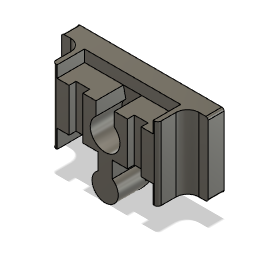
Duplo_Eisenbahn_adapter (Autodesk Fusion 360 design; units mm, degrees)
Autodesk Fusion 360 part; units mm, degrees
note: some values were not read from the file. Set by a fixed rule: which sketch regions a step uses.
sketch "Skizze1" plane through (0, 0, 0) normal (0, 0, 1) x (1, 0, 0)
  line L0 (32, 16) -> (-32, 16)
  line L1 (-32, 16) -> (-32, -16)
  line L2 (-32, -16) -> (32, -16)
  line L3 (32, -16) -> (32, 16)
  line L4 (32, 16) -> (-32, -16) construction
  line L5 (-32, 16) -> (32, -16) construction
  dimension "d1" = 64
  dimension "d2" = 32
  constraint horizontal L0
  constraint perpendicular L0 L1
  constraint parallel L0 L2
  constraint parallel L1 L3
  constraint coincident L4 origin
  constraint coincident L5 origin
  measures "d1" distance of L1.end L2.end
  measures "d2" distance of L0.end L1.end
extrude "Extrusion1" add sketch "Skizze1" along normal blind 20
sketch "Skizze2" plane through (0, 0, 0) normal (0, 0, -1) x (-1, 0, 0)
  line L0 (-32, 16) -> (-32, -16)
  line L1 (-32, -16) -> (32, -16)
  line L2 (32, -16) -> (32, 16)
  line L3 (32, 16) -> (-32, 16)
  line L4 (30.25, 14.25) -> (-30.25, 14.25)
  line L5 (-30.25, 14.25) -> (-30.25, -14.25)
  line L6 (-30.25, -14.25) -> (30.25, -14.25)
  line L7 (30.25, -14.25) -> (30.25, 14.25)
  line L8 (30.25, 14.25) -> (-30.25, -14.25) construction
  line L9 (-30.25, 14.25) -> (30.25, -14.25) construction
  line L10 (-25, 14.25) -> (-23.5, 14.25)
  line L11 (-23.5, 14.25) -> (-23.5, 12.75)
  line L12 (-23.5, 12.75) -> (-25, 12.75)
  line L13 (-25, 12.75) -> (-25, 14.25)
  line L14 (-30.25, 9) -> (-28.75, 9)
  line L15 (-28.75, 9) -> (-28.75, 7.5)
  line L16 (-28.75, 7.5) -> (-30.25, 7.5)
  line L17 (-30.25, 7.5) -> (-30.25, 9)
  line L18 (-10, 14.25) -> (-8.5, 14.25)
  line L19 (-8.5, 14.25) -> (-8.5, 12.75)
  line L20 (-8.5, 12.75) -> (-10, 12.75)
  line L21 (-10, 12.75) -> (-10, 14.25)
  line L22 (-24.25, 12.75) -> (-24.25, 14.25) construction
  line L23 (-28.75, 8.25) -> (-30.25, 8.25) construction
  line L24 (-9.25, 12.75) -> (-9.25, 14.25) construction
  line L25 (0, 0) -> (0, 14.25) construction
  line L26 (0, 0) -> (-30.25, 0) construction
  line L27 (24.25, 12.75) -> (24.25, 14.25) construction
  line L28 (8.5, 14.25) -> (8.5, 12.75)
  line L29 (28.75, 7.5) -> (30.25, 7.5)
  line L30 (10, 14.25) -> (8.5, 14.25)
  line L31 (8.5, 12.75) -> (10, 12.75)
  line L32 (23.5, 12.75) -> (25, 12.75)
  line L33 (28.75, 8.25) -> (30.25, 8.25) construction
  line L34 (28.75, 9) -> (28.75, 7.5)
  line L35 (25, 12.75) -> (25, 14.25)
  line L36 (30.25, 7.5) -> (30.25, 9)
  line L37 (9.25, 12.75) -> (9.25, 14.25) construction
  line L38 (30.25, 9) -> (28.75, 9)
  line L39 (10, 12.75) -> (10, 14.25)
  line L40 (25, 14.25) -> (23.5, 14.25)
  line L41 (23.5, 14.25) -> (23.5, 12.75)
  line L42 (-25, -12.75) -> (-25, -14.25)
  line L43 (-28.75, -9) -> (-28.75, -7.5)
  line L44 (-30.25, -9) -> (-28.75, -9)
  line L45 (30.25, -14.25) -> (-30.25, -14.25)
  line L46 (-28.75, -8.25) -> (-30.25, -8.25) construction
  line L47 (25, -14.25) -> (23.5, -14.25)
  line L48 (-10, -14.25) -> (-8.5, -14.25)
  line L49 (23.5, -12.75) -> (25, -12.75)
  line L50 (-23.5, -14.25) -> (-23.5, -12.75)
  line L51 (32, -16) -> (-32, -16)
  line L52 (10, -12.75) -> (10, -14.25)
  line L53 (-9.25, -12.75) -> (-9.25, -14.25) construction
  line L54 (-28.75, -7.5) -> (-30.25, -7.5)
  line L55 (8.5, -12.75) -> (10, -12.75)
  line L56 (-10, -12.75) -> (-10, -14.25)
  line L57 (28.75, -8.25) -> (30.25, -8.25) construction
  line L58 (-25, -14.25) -> (-23.5, -14.25)
  line L59 (8.5, -14.25) -> (8.5, -12.75)
  line L60 (24.25, -12.75) -> (24.25, -14.25) construction
  line L61 (-23.5, -12.75) -> (-25, -12.75)
  line L62 (30.25, -9) -> (28.75, -9)
  line L63 (-8.5, -14.25) -> (-8.5, -12.75)
  line L64 (23.5, -14.25) -> (23.5, -12.75)
  line L65 (30.25, -7.5) -> (30.25, -9)
  line L66 (10, -14.25) -> (8.5, -14.25)
  line L67 (-24.25, -12.75) -> (-24.25, -14.25) construction
  line L68 (28.75, -9) -> (28.75, -7.5)
  line L69 (9.25, -12.75) -> (9.25, -14.25) construction
  line L70 (-8.5, -12.75) -> (-10, -12.75)
  line L71 (-30.25, -7.5) -> (-30.25, -9)
  line L72 (28.75, -7.5) -> (30.25, -7.5)
  line L73 (25, -12.75) -> (25, -14.25)
  circle A0 centre (0, 0) radius 6.575
  circle A1 centre (16, 0) radius 6.575
  circle A2 centre (-16, 0) radius 6.575
  circle A3 centre (-16, 0) radius 5.075
  circle A4 centre (0, 0) radius 5.075
  circle A5 centre (16, 0) radius 5.075
  point P0 (32, 16)
  point P1 (30.25, 14.25)
  point P2 (0, -14.25)
  point P3 (32, -16)
  point P4 (30.25, -14.25)
  dimension "d7" = 1.75
  dimension "d8" = 1.75
  dimension "d9" = 1.5
  dimension "d10" = 1.5
  dimension "d11" = 6
  dimension "d12" = 6
  dimension "d13" = 15
  dimension "d14" = 13.15
  dimension "d17" = 16
  dimension "d18" = 0
  dimension "d19" = 1.5
  constraint horizontal L4
  constraint perpendicular L4 L5
  constraint parallel L4 L6
  constraint parallel L5 L7
  constraint coincident L8 L25.start
  constraint coincident L9 L25.start
  constraint coincident L25.start L26.start
  constraint horizontal L10
  constraint vertical L11
  constraint horizontal L12
  constraint vertical L13
  constraint coincident L4 L10.start
  constraint horizontal L14
  constraint vertical L15
  constraint horizontal L16
  constraint vertical L17
  constraint coincident L5 L14.start
  constraint horizontal L18
  constraint vertical L19
  constraint horizontal L20
  constraint vertical L21
  constraint coincident L4 L18.start
  constraint collinear L12 L20
  constraint equal L13 L14
  constraint equal L12 L20
  constraint equal L12 L15
  constraint midpoint L12 L22.start
  constraint midpoint L10 L22.end
  constraint midpoint L15 L23.start
  constraint midpoint L17 L23.end
  constraint midpoint L20 L24.start
  constraint midpoint L18 L24.end
  constraint midpoint L4 L25.end
  constraint midpoint L5 L26.end
  constraint symmetric L0.start L25 P0
  constraint symmetric L4.end L25 P1
  constraint symmetric L10.start L25 L35.end
  constraint symmetric L10.end L25 L40.end
  constraint symmetric L11.end L25 L32.start
  constraint symmetric L12.end L25 L32.end
  constraint symmetric L14.start L25 L36.end
  constraint symmetric L14.end L25 L34.start
  constraint symmetric L15.end L25 L29.start
  constraint symmetric L16.end L25 L29.end
  constraint symmetric L18.start L25 L30.start
  constraint symmetric L18.end L25 L28.start
  constraint symmetric L19.end L25 L28.end
  constraint symmetric L20.end L25 L31.end
  constraint symmetric L22.start L25 L27.start
  constraint symmetric L22.end L25 L27.end
  constraint symmetric L23.start L25 L33.start
  constraint symmetric L23.end L25 L33.end
  constraint symmetric L24.start L25 L37.start
  constraint symmetric L24.end L25 L37.end
  constraint symmetric L0.start L26 L0.end
  constraint symmetric P0 L26 P3
  constraint symmetric P1 L26 P4
  constraint symmetric L4.end L26 L5.end
  constraint symmetric L10.start L26 L42.end
  constraint symmetric L10.end L26 L50.start
  constraint symmetric L11.end L26 L50.end
  constraint symmetric L12.end L26 L42.start
  constraint symmetric L14.start L26 L44.start
  constraint symmetric L14.end L26 L43.start
  constraint symmetric L15.end L26 L43.end
  constraint symmetric L16.end L26 L54.end
  constraint symmetric L18.start L26 L48.start
  constraint symmetric L18.end L26 L48.end
  constraint symmetric L19.end L26 L63.end
  constraint symmetric L20.end L26 L56.start
  constraint symmetric L22.start L26 L67.start
  constraint symmetric L22.end L26 L67.end
  constraint symmetric L23.start L26 L46.start
  constraint symmetric L23.end L26 L46.end
  constraint symmetric L24.start L26 L53.start
  constraint symmetric L24.end L26 L53.end
  constraint symmetric L25.end L26 P2
  constraint symmetric L26 L40.end L47.end
  constraint symmetric L26 L28.start L59.start
  constraint symmetric L26 L30.start L52.end
  constraint symmetric L26 L37.start L69.start
  constraint symmetric L26 L33.end L57.end
  constraint symmetric L26 L37.end L69.end
  constraint symmetric L26 L29.end L65.start
  constraint symmetric L26 L29.start L68.end
  constraint symmetric L26 P0 P3
  constraint symmetric L26 L36.end L62.start
  constraint symmetric L26 L34.start L62.end
  constraint symmetric L26 L28.end L55.start
  constraint symmetric L26 L33.start L57.start
  constraint symmetric L26 L27.end L60.end
  constraint symmetric L26 L27.start L60.start
  constraint symmetric L26 L31.end L52.start
  constraint symmetric L26 L32.start L49.start
  constraint symmetric L26 L32.end L49.end
  constraint symmetric L26 L35.end L47.start
  constraint symmetric L26 P1 P4
  constraint concentric A2 A3
  constraint concentric A1 A5
  constraint equal A4 A5
  constraint equal A3 A4
  measures "d7" distance of L3 L4
  measures "d8" distance of L0 L5
  measures "d9" distance of L10.end L11.end
  measures "d10" distance of L11.end L12.end
  measures "d11" distance of L4 L23
  measures "d12" distance of L5 L22
  measures "d13" distance of L22 L24
  measures "d14" diameter of A0
  measures "d19" distance of A1 A5
extrude "Extrusion2" cut sketch "Skizze2" against normal blind 5 contours L4 L5 L6 L7 L11 L12 L13 L14 L15 L16 L19 L20 L21 L28 L29 L31 L32 L34 L35 L38 L39 L41 L42 L43 L44 L45 L49 L50 L52 L54 L55 L56 L59 L61 L62 L63 L64 L68 L70 L72 L73 | A3 | A4 | A5
sketch "Skizze3" plane through (0, 0, 20) normal (0, 0, 1) x (1, 0, 0)
  line L0 (32, -16) -> (32, 16)
  line L1 (32, 16) -> (-32, 16)
  line L2 (-32, 16) -> (-32, -16)
  line L3 (-32, -16) -> (32, -16)
  circle A0 centre (0, -0.1235) radius 6.5
  line L4 (0, -0.1235) -> (0, 16) construction
  line L5 (-21, 16) -> (21, 16)
  line L6 (21, 16) -> (21, 10.8765)
  line L7 (21, 10.8765) -> (-21, 10.8765)
  line L8 (-21, 10.8765) -> (-21, 16)
  line L9 (-21, 16) -> (21, 10.8765) construction
  line L10 (21, 16) -> (-21, 10.8765) construction
  line L11 (-4, 5) -> (4, 5)
  line L12 (4, 5) -> (4, 10.8765)
  line L13 (4, 10.8765) -> (-4, 10.8765)
  line L14 (-4, 10.8765) -> (-4, 5)
  line L15 (-4, 5) -> (4, 10.8765) construction
  line L16 (4, 5) -> (-4, 10.8765) construction
  point P0 (0, 13.4383)
  point P1 (0, 7.9383)
  dimension "d22" = 42
  dimension "d23" = 8
  dimension "d24" = 13
  dimension "d25" = 11
  constraint coincident A0.centre L4.start
  constraint midpoint L1 L4.end
  constraint horizontal L5
  constraint perpendicular L5 L6
  constraint parallel L5 L7
  constraint parallel L6 L8
  constraint coincident L9 P0
  constraint coincident L10 P0
  constraint coincident L1 L5.start
  constraint coincident L4 P0
  constraint horizontal L11
  constraint perpendicular L11 L12
  constraint parallel L11 L13
  constraint parallel L12 L14
  constraint coincident L15 P1
  constraint coincident L16 P1
  constraint coincident A0 L11.start
  constraint midpoint L4 P1
  constraint collinear L7 L13
  constraint coincident origin L4
  measures "d22" distance of L6.end L7.end
  measures "d23" distance of L12 L14
  measures "d24" diameter of A0
  measures "d25" distance of A0.centre L7
extrude "Extrusion3" cut sketch "Skizze3" against normal blind 12 contours L1 L5 L6 L7 L8 L13 | A0 L7 L12 L13 L14 | A0 L11 | A0 L11
sketch "Skizze4" plane through (0, 0, 20) normal (0, 0, 1) x (1, 0, 0)
  line L0 (-21, 10.8765) -> (-21, 16)
  line L1 (-21, 16) -> (-32, 16)
  line L2 (-32, 16) -> (-32, -16)
  line L3 (-32, -16) -> (32, -16)
  line L4 (32, -16) -> (32, 16)
  line L5 (32, 16) -> (21, 16)
  line L6 (21, 16) -> (21, 10.8765)
  line L7 (21, 10.8765) -> (4, 10.8765)
  line L8 (4, 10.8765) -> (4, 5)
  arc A0 (-4, 5) -> (4, 5) centre (0, -0.1235) ccw
  line L9 (-4, 5) -> (-4, 10.8765)
  line L10 (-4, 10.8765) -> (-21, 10.8765)
  line L11 (0, 0) -> (0, -20) construction
  circle A1 centre (0, -20) radius 5.75
  line L12 (-3.1, -15.1572) -> (3.1, -15.1572)
  line L13 (3.1, -15.1572) -> (3.1, -8)
  line L14 (3.1, -8) -> (-3.1, -8)
  line L15 (-3.1, -8) -> (-3.1, -15.1572)
  line L16 (-3.1, -15.1572) -> (3.1, -8) construction
  line L17 (3.1, -15.1572) -> (-3.1, -8) construction
  line L18 (-21, -8) -> (21, -8)
  line L19 (21, -8) -> (21, -28)
  line L20 (21, -28) -> (-21, -28)
  line L21 (-21, -28) -> (-21, -8)
  line L22 (-21, -8) -> (21, -28) construction
  line L23 (21, -8) -> (-21, -28) construction
  point P0 (0, -11.5786)
  point P1 (0, -18)
  dimension "d29" = 11.5
  dimension "d30" = 6.2
  dimension "d31" = 8
  dimension "d32" = 12
  dimension "d33" = 20
  dimension "d34" = 42
  constraint coincident L11.start origin
  constraint vertical L11
  constraint coincident L11.end A1.centre
  constraint horizontal L12
  constraint perpendicular L12 L13
  constraint parallel L12 L14
  constraint parallel L13 L15
  constraint coincident L16 P0
  constraint coincident L17 P0
  constraint coincident A1 L12.start
  constraint coincident L11 P0
  constraint horizontal L18
  constraint perpendicular L18 L19
  constraint parallel L18 L20
  constraint parallel L19 L21
  constraint coincident L22 P1
  constraint coincident L23 P1
  constraint coincident L11 P1
  constraint collinear L14 L18
  measures "d29" diameter of A1
  measures "d30" distance of L13.end L14.end
  measures "d31" distance of L11.start L18
  measures "d32" distance of L11.end L18
  measures "d33" distance of L18.start L20.end
  measures "d34" distance of L19.end L20.end
extrude "Extrusion4" cut sketch "Skizze4" against normal blind 12 contours L3 A1 L15 L18 L21 | L3 A1 L13 L18 L19
extrude "Extrusion5" add sketch "Skizze4" against normal blind 20 contours L3 A1
fillet "Abrundung1" radius 5 2 edges at (-4.1307, -16, 4) (4.1307, -16, 4)
sketch "Skizze5" plane through (0, 0, 20) normal (0, 0, 1) x (1, 0, 0)
  line L0 (21, -8) -> (21, -16)
  line L1 (21, -16) -> (32, -16)
  line L2 (32, -16) -> (32, 16)
  line L3 (32, 16) -> (21, 16)
  line L4 (21, 16) -> (21, 10.8765)
  line L5 (21, 10.8765) -> (4, 10.8765)
  line L6 (4, 10.8765) -> (4, 5)
  arc A0 (-4, 5) -> (4, 5) centre (0, -0.1235) ccw
  line L7 (-4, 5) -> (-4, 10.8765)
  line L8 (-4, 10.8765) -> (-21, 10.8765)
  line L9 (-21, 10.8765) -> (-21, 16)
  line L10 (-21, 16) -> (-32, 16)
  line L11 (-32, 16) -> (-32, -16)
  line L12 (-32, -16) -> (-21, -16)
  line L13 (-21, -16) -> (-21, -8)
  line L14 (-21, -8) -> (-3.1, -8)
  line L15 (-3.1, -8) -> (-3.1, -15.1572)
  arc A1 (-3.1, -15.1572) -> (3.1, -15.1572) centre (0, -20) ccw
  line L16 (3.1, -15.1572) -> (3.1, -8)
  line L17 (3.1, -8) -> (21, -8)
  line L18 (0, -0.1235) -> (0, 16)
  line L19 (-9.75, 16) -> (-15.75, 16)
  line L20 (-15.75, 16) -> (-15.75, -16)
  line L21 (-15.75, -16) -> (-9.75, -16)
  line L22 (-9.75, -16) -> (-9.75, 16)
  line L23 (9.75, 16) -> (15.75, 16)
  line L24 (15.75, 16) -> (15.75, -16)
  line L25 (15.75, -16) -> (9.75, -16)
  line L26 (9.75, -16) -> (9.75, 16)
  dimension "d41" = 6
  dimension "d42" = 19.5
  constraint coincident A0.centre L18.start
  constraint vertical L18
  constraint horizontal L19
  constraint vertical L20
  constraint horizontal L21
  constraint vertical L22
  constraint horizontal L23
  constraint vertical L24
  constraint horizontal L25
  constraint vertical L26
  measures "d41" distance of L19.start L19.end
  measures "d42" distance of L22 L26
extrude "Extrusion6" cut sketch "Skizze5" against normal blind 3 contours L5 L17 L24 L26 | L8 L14 L20 L22
sketch "Skizze7" plane through (32, 0, 0) normal (1, 0, 0) x (0, 0, -1)
  line L0 (-20, -16) -> (0, -16)
  line L1 (0, -16) -> (0, 16)
  line L2 (0, 16) -> (-20, 16)
  line L3 (0, -16) -> (-11.3908, -27)
  line L4 (-11.3908, -27) -> (0, -27)
  line L5 (0, -27) -> (0, -16)
  line L6 (-20, 16) -> (-20, -16)
  dimension "d46" = 11
  dimension "d49" = 46
  constraint coincident L0.end L1.start
  constraint perpendicular L1 L4
  constraint perpendicular L0 L5
  measures "d46" distance of L4.end L0.end
  measures "d49" angle of L3 L5
extrude "Extrusion7" cut sketch "Skizze7" against normal blind 64 contours L3 L4 L5
ref_plane "Arbeitsebene1" through (-12.5, 10.8765, 8) normal (0, -0.173648, 0.984808) x (-1, 0, 0)
sketch "Skizze8" plane through (0, 0, 8) normal (0, 0, 1) x (1, 0, 0)
  line L0 (-21, 10.8765) -> (-4, 10.8765)
  line L1 (-4, 10.8765) -> (-4, 5)
  arc A0 (-4, 5) -> (4, 5) centre (0, -0.1235) ccw
  line L2 (4, 5) -> (4, 10.8765)
  line L3 (4, 10.8765) -> (21, 10.8765)
  line L4 (21, 10.8765) -> (21, 16)
  line L5 (21, 16) -> (-21, 16)
  line L6 (-21, 16) -> (-21, 10.8765)
  line L7 (-4, 10.8765) -> (4, 10.8765)
  constraint coincident L0.end L1.start
  constraint coincident L2.end L3.start
extrude "Extrusion8" cut sketch "Skizze8" along normal up to surface contours L1 A0 L2 L7 end surface through (-12.5, 10.8765, 8) normal (0, -0.173648, 0.984808) offset 0
sketch "Skizze9" plane through (0, 16, 0) normal (0, 1, 0) x (-1, 0, 0)
  line L0 (21, 20) -> (21, 8)
  line L1 (21, 8) -> (-21, 8)
  line L2 (-21, 8) -> (-21, 20)
  line L3 (-21, 20) -> (-32, 20)
  line L4 (-32, 20) -> (-32, 0)
  line L5 (-32, 0) -> (32, 0)
  line L6 (32, 0) -> (32, 20)
  line L7 (32, 20) -> (21, 20)
  line L8 (23.5, 5) -> (25, 5)
  line L9 (25, 5) -> (30.25, 5)
  line L10 (30.25, 5) -> (28.75, 5)
  line L11 (28.75, 5) -> (30.25, 5)
  line L12 (30.25, 5) -> (28.75, 5)
  line L13 (28.75, 5) -> (30.25, 5)
  line L14 (30.25, 5) -> (25, 5)
  line L15 (25, 5) -> (23.5, 5)
  line L16 (23.5, 5) -> (10, 5)
  line L17 (10, 5) -> (8.5, 5)
  line L18 (8.5, 5) -> (-8.5, 5)
  line L19 (-8.5, 5) -> (-10, 5)
  line L20 (-10, 5) -> (-23.5, 5)
  line L21 (-23.5, 5) -> (-25, 5)
  line L22 (-25, 5) -> (-30.25, 5)
  line L23 (-30.25, 5) -> (-28.75, 5)
  line L24 (-28.75, 5) -> (-30.25, 5)
  line L25 (-30.25, 5) -> (-28.75, 5)
  line L26 (-28.75, 5) -> (-30.25, 5)
  line L27 (-30.25, 5) -> (-25, 5)
  line L28 (-25, 5) -> (-23.5, 5)
  line L29 (-23.5, 5) -> (-10, 5)
  line L30 (-10, 5) -> (-8.5, 5)
  line L31 (-8.5, 5) -> (8.5, 5)
  line L32 (8.5, 5) -> (10, 5)
  line L33 (10, 5) -> (23.5, 5)
  line L34 (9.425, 5) -> (22.575, 5)
  line L35 (-22.575, 5) -> (-9.425, 5)
  line L36 (2.3588, 5) -> (2.4665, 5)
  line L37 (2.4665, 5) -> (-2.4665, 5)
  line L38 (-2.4665, 5) -> (-2.3588, 5)
  line L39 (-6.575, 5) -> (6.575, 5)
  line L40 (-32, 7) -> (-23, 7)
  line L41 (-23, 7) -> (-23, 20)
  line L42 (-23, 20) -> (-32, 20)
  line L43 (-32, 20) -> (-32, 7)
  line L44 (32, 20) -> (23, 20)
  line L45 (23, 20) -> (23, 7)
  line L46 (23, 7) -> (32, 7)
  line L47 (32, 7) -> (32, 20)
  dimension "d55" = 2
  dimension "d56" = 2
  dimension "d57" = 2
  constraint horizontal L40
  constraint vertical L41
  constraint horizontal L42
  constraint vertical L43
  constraint coincident L3 L41.end
  constraint horizontal L44
  constraint vertical L45
  constraint horizontal L46
  constraint vertical L47
  constraint coincident L6.end L7.start
  constraint collinear L40 L46
  measures "d55" distance of L2 L41
  measures "d56" distance of L27 L40
  measures "d57" distance of L0 L45
extrude "Extrusion9" cut sketch "Skizze9" against normal blind 32 contours L6 L7 L44 L45 L46 L47 | L3 L4 L40 L41 L42 L43
fillet "Abrundung2" radius 5 2 edges at (-23, 0, 7) (23, 0, 7)
fillet "Abrundung3" radius 1.5 2 edges at (23, 0, 20) (-23, 0, 20)
fillet "Abrundung4" radius 1 4 edges at (-32, 16, 3.5) (-32, -16, 3.5) (32, 16, 3.5) (32, -16, 3.5)
equation "d8 = d7"
equation "d12 = d11"
equation "d56 = d55"
equation "d57 = d55"
